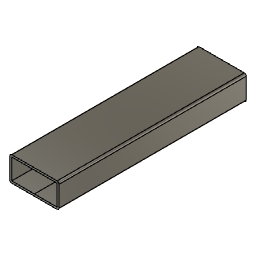
_Profil50x25_190mm.0e040478-a610-48e4-aa6a-0250c9300f2e (Autodesk Fusion 360 design; units mm, degrees)
Autodesk Fusion 360 part; units mm, degrees
sketch "Sketch1" plane through (0, 0, 0) normal (0, 1, 0) x (1, 0, 0)
  line L0 (0, -12.5) -> (23, -12.5)
  line L1 (25, -10.5) -> (25, 10.5)
  line L2 (23, 12.5) -> (0, 12.5)
  line L3 (0, -12.5) -> (-23, -12.5)
  line L4 (-25, -10.5) -> (-25, 10.5)
  line L5 (-23, 12.5) -> (0, 12.5)
  arc A0 (-25, -10.5) -> (-23, -12.5) centre (-23, -10.5) ccw
  arc A1 (23, -12.5) -> (25, -10.5) centre (23, -10.5) ccw
  arc A2 (-23, 12.5) -> (-25, 10.5) centre (-23, 10.5) ccw
  line L6 (-23, 10.5) -> (0, 10.5)
  line L7 (23, 10.5) -> (0, 10.5)
  line L8 (23, -10.5) -> (23, 10.5)
  line L9 (0, -10.5) -> (23, -10.5)
  line L10 (0, -10.5) -> (-23, -10.5)
  line L11 (-23, -10.5) -> (-23, 10.5)
  arc A3 (25, 10.5) -> (23, 12.5) centre (23, 10.5) ccw
  point P0 (25, -12.5)
  dimension "d1" = 12.5
  dimension "d2" = 25
  dimension "d3" = 25
  dimension "d4" = 2
  dimension "d5" = 2
  dimension "d6" = 2
  dimension "d7" = 2
  constraint horizontal L0
  constraint vertical L1
  constraint horizontal L2
  constraint tangent L3 A0
  constraint tangent L4 A0
  constraint coincident P0 L0
  constraint coincident P0 L1
  constraint tangent L0 A1
  constraint tangent L1 A1
  constraint tangent L4 A2
  constraint tangent L5 A2
  constraint tangent L1 A3
  constraint tangent L2 A3
  constraint equal A2 A3
  measures "d1" distance of origin L0.start
  measures "d2" distance of L0.start P0
  measures "d3" distance of L0.start L2.end
  measures "d5" radius of A0
  measures "d6" radius of A1
  measures "d7" radius of A2
extrude "Extrude2" add sketch "Sketch1" along normal blind 190
